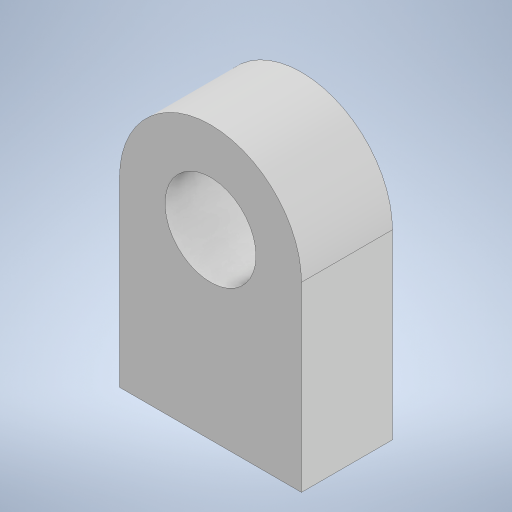
# Autodesk Inventor part: gối
Saved by Autodesk Inventor 2024 (Build 280153000, 153)
## iProperties
Created: 2025-09-18
Part Number: gối
Material: Generic
Document SubType Name: Modeling
Designer: Hello
Density: 1 g/cm^3
Appearance: Default
Author: Hello
Autodesk Inventor part; units mm, degrees
ref_plane "YZ Plane" through (0, 0, 0) normal (1, 0, 0) x (0, 1, 0)
ref_plane "XZ Plane" through (0, 0, 0) normal (0, 1, 0) x (-1, 0, 0)
ref_plane "XY Plane" through (0, 0, 0) normal (0, 0, 1) x (1, 0, 0)
sketch "Sketch1" plane through (0, 0, 0) normal (0, 0, 1) x (1, 0, 0)
  line L0 (0, 0) -> (20, 0)
  line L1 (20, 0) -> (20, 20)
  line L2 (0, 20) -> (0, 0)
  arc A0 (20, 20) -> (0, 20) centre (10, 20) ccw
  circle A1 centre (10, 20) radius 5
  dimension "d0" = 20
  dimension "d1" = 20
  dimension "d2" = 10
  constraints: 6 end point, 2 centre point, 2 point on circle, 1 coincident, 1 horizontal, 1 parallel, 1 perpendicular, 1 tangent
  measures "d0" distance of L2.start L0.start
  measures "d1" distance of L0.start L0.end
  measures "d2" diameter of A1
extrude "Extrusion1" add sketch "Sketch1" along normal blind 10
body "Solid1"
